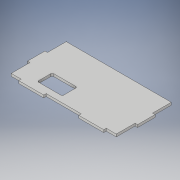
# Autodesk Inventor part: Part Sisi 1
Saved by Autodesk Inventor 2019 (Build 230136000, 136)
## iProperties
Created: 2019-07-08
Part Number: Part Sisi 1
Material: Generic
Document SubType Name: Modeling
Designer: azriel
Density: 1 g/cm^3
Appearance: Default
Author: azriel
Autodesk Inventor part; units mm, degrees
ref_plane "YZ Plane" through (0, 0, 0) normal (1, 0, 0) x (0, 1, 0)
ref_plane "XZ Plane" through (0, 0, 0) normal (0, 1, 0) x (-1, 0, 0)
ref_plane "XY Plane" through (0, 0, 0) normal (0, 0, 1) x (1, 0, 0)
sketch "Sketch1" plane through (0, 0, 0) normal (0, 1, 0) x (-1, 0, 0)
  line L0 (4.6863, 62.0394) -> (4.6863, 67.0394)
  line L1 (54.6863, 67.0394) -> (54.6863, 62.0394)
  line L2 (74.6863, 62.0394) -> (54.6863, 62.0394)
  line L3 (-65.3137, 62.0394) -> (-65.3137, 67.0394)
  line L4 (-115.3137, 67.0394) -> (-115.3137, 62.0394)
  line L5 (4.6863, 62.0394) -> (-65.3137, 62.0394)
  line L6 (-115.3137, 62.0394) -> (-135.3137, 62.0394)
  line L7 (-135.3137, -47.9606) -> (-115.3137, -47.9606)
  line L8 (-65.3137, -47.9606) -> (4.6863, -47.9606)
  line L9 (54.6863, -47.9606) -> (74.6863, -47.9606)
  line L10 (79.6863, -10.4606) -> (74.6863, -10.4606)
  line L11 (74.6863, -10.4606) -> (74.6863, -47.9606)
  line L12 (79.6863, -10.4606) -> (79.6863, 24.5394)
  line L13 (79.6863, 24.5394) -> (74.6863, 24.5394)
  line L14 (74.6863, 24.5394) -> (74.6863, 62.0394)
  line L15 (-140.3137, -10.4606) -> (-140.3137, 24.5394)
  line L16 (-140.3137, -10.4606) -> (-135.3137, -10.4606)
  line L17 (-135.3137, -10.4606) -> (-135.3137, -47.9606)
  line L18 (-140.3137, 24.5394) -> (-135.3137, 24.5394)
  line L19 (-135.3137, 24.5394) -> (-135.3137, 62.0394)
  line L20 (31.6863, 50.0394) -> (-12.3137, 50.0394)
  line L21 (-15.3137, 47.0394) -> (-15.3137, 23.0394)
  line L22 (-12.3137, 20.0394) -> (31.6863, 20.0394)
  line L23 (34.6863, 23.0394) -> (34.6863, 47.0394)
  arc A0 (31.6863, 20.0394) -> (34.6863, 23.0394) centre (31.6863, 23.0394) ccw
  arc A1 (34.6863, 47.0394) -> (31.6863, 50.0394) centre (31.6863, 47.0394) ccw
  arc A2 (-12.3137, 50.0394) -> (-15.3137, 47.0394) centre (-12.3137, 47.0394) ccw
  arc A3 (-15.3137, 23.0394) -> (-12.3137, 20.0394) centre (-12.3137, 23.0394) ccw
  line L24 (54.6863, -47.9606) -> (-115.3137, -47.9606)
  line L25 (4.6863, 62.0394) -> (4.6863, 67.0394)
  line L26 (4.6863, 67.0394) -> (54.6863, 67.0394)
  line L27 (-65.3137, 67.0394) -> (-115.3137, 67.0394)
  point P0 (0, 0)
  point P1 (34.6863, 50.0394)
  point P2 (-15.3137, 50.0394)
  point P3 (-15.3137, 20.0394)
  dimension "d6" = 50
  dimension "d12" = 70
  dimension "d40" = 50
  dimension "d41" = 30
  dimension "d44" = 5
  dimension "d46" = 3
  dimension "d49" = 5
  constraints: 56 end point, 13 parallel, 8 perpendicular, 8 point on circle, 8 point on line, 8 tangent, 4 centre point, 4 horizontal, 3 equal radius, 1 vertical
  measures "d6" distance of L1.end L0.start
  measures "d12" distance between parallel lines of L3 L0
  measures "d40" distance of point (34.686, 50.039) point (-15.314, 50.039)
  measures "d41" distance of point (-15.314, 20.039) point (-15.314, 50.039)
  measures "d44" distance of L13.end L12.end
  measures "d46" radius of A0
  measures "d49" distance of L0.end L0.start
extrude "Extrusion3" add sketch "Sketch1" along normal blind 5
body "Solid3"
